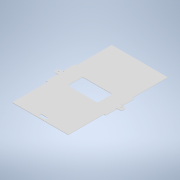
# Autodesk Inventor part: metal_body_forPrint
Saved by Autodesk Inventor 2022 (Build 260153000, 153)
## iProperties
Created: 2024-12-12
Part Number: metal_body_forPrint
Material: Типовые
Document SubType Name: Modeling
Designer: Andrey
Density: 1 g/cm^3
Appearance: По умолчанию
Author: Andrey
Autodesk Inventor part; units mm, degrees
ref_plane "YZ Plane" through (0, 0, 0) normal (1, 0, 0) x (0, 1, 0)
ref_plane "XZ Plane" through (0, 0, 0) normal (0, 1, 0) x (-1, 0, 0)
ref_plane "XY Plane" through (0, 0, 0) normal (0, 0, 1) x (1, 0, 0)
sketch "Эскиз1" plane through (0, 0, 0) normal (0, 1, 0) x (-1, 0, 0)
  line L0 (42.275, -3.8) -> (42.275, -4.36)
  arc A0 (40.675, -5.96) -> (42.275, -4.36) centre (40.675, -4.36) ccw
  line L1 (40.675, -5.96) -> (34.325, -5.96)
  arc A1 (32.725, -4.36) -> (34.325, -5.96) centre (34.325, -4.36) ccw
  line L2 (32.725, -4.36) -> (32.725, -3.8)
  arc A2 (34.325, -2.2) -> (32.725, -3.8) centre (34.325, -3.8) ccw
  line L3 (34.325, -2.2) -> (40.675, -2.2)
  arc A3 (42.275, -3.8) -> (40.675, -2.2) centre (40.675, -3.8) ccw
  arc A4 (55.5, -76.631) -> (57.5, -74.631) centre (55.5, -74.631) ccw
  line L4 (55.5, -76.631) -> (19.5, -76.631)
  arc A5 (17.5, -74.631) -> (19.5, -76.631) centre (19.5, -74.631) ccw
  line L5 (17.5, -74.631) -> (17.5, -58.631)
  arc A6 (19.5, -56.631) -> (17.5, -58.631) centre (19.5, -58.631) ccw
  line L6 (19.5, -56.631) -> (55.5, -56.631)
  arc A7 (57.5, -58.631) -> (55.5, -56.631) centre (55.5, -58.631) ccw
  line L7 (57.5, -58.631) -> (57.5, -74.631)
  line L8 (77.5, -85.631) -> (75, -85.631)
  line L9 (75, -47.631) -> (77.5, -47.631)
  line L10 (75, -47.631) -> (75, 0)
  line L11 (75, 0) -> (0, 0)
  line L12 (0, -47.631) -> (0, 0)
  line L13 (-2.5, -47.631) -> (0, -47.631)
  line L14 (0, -85.631) -> (-2.5, -85.631)
  line L15 (0, -85.631) -> (0, -133.2619)
  line L16 (0, -133.2619) -> (75, -133.2619)
  line L17 (75, -85.631) -> (75, -133.2619)
  line L18 (-0.95, -70.631) -> (-2.5, -70.631)
  line L19 (-2.5, -85.631) -> (-2.5, -70.631)
  line L20 (-2.5, -62.631) -> (-2.5, -47.631)
  line L21 (-2.5, -62.631) -> (-0.95, -62.631)
  line L22 (-0.95, -62.631) -> (-0.95, -63.131)
  line L23 (-4.831, -63.131) -> (-0.95, -63.131)
  line L24 (-4.831, -70.131) -> (-0.95, -70.131)
  line L25 (-0.95, -70.131) -> (-0.95, -70.631)
  arc A8 (-4.831, -63.131) -> (-4.831, -70.131) centre (-4.831, -66.631) ccw
  line L26 (77.5, -70.631) -> (77.5, -85.631)
  line L27 (77.5, -70.631) -> (75.95, -70.631)
  line L28 (75.95, -70.631) -> (75.95, -70.131)
  line L29 (79.831, -70.131) -> (75.95, -70.131)
  arc A9 (79.831, -70.131) -> (79.831, -63.131) centre (79.831, -66.631) ccw
  line L30 (79.831, -63.131) -> (75.95, -63.131)
  line L31 (75.95, -63.131) -> (75.95, -62.631)
  line L32 (75.95, -62.631) -> (77.5, -62.631)
  line L33 (77.5, -47.631) -> (77.5, -62.631)
  arc A10 (55.5, -76.631) -> (57.5, -74.631) centre (55.5, -74.631) ccw
  line L34 (57.5, -74.631) -> (57.5, -58.631)
  arc A11 (57.5, -58.631) -> (55.5, -56.631) centre (55.5, -58.631) ccw
  line L35 (55.5, -56.631) -> (19.5, -56.631)
  arc A12 (19.5, -56.631) -> (17.5, -58.631) centre (19.5, -58.631) ccw
  line L36 (17.5, -58.631) -> (17.5, -74.631)
  arc A13 (17.5, -74.631) -> (19.5, -76.631) centre (19.5, -74.631) ccw
  line L37 (19.5, -76.631) -> (55.5, -76.631)
  circle A14 centre (79.831, -66.631) radius 1
  circle A15 centre (-4.831, -66.631) radius 1
  line L38 (42.275, -4.36) -> (42.275, -3.8)
  arc A16 (42.275, -3.8) -> (40.675, -2.2) centre (40.675, -3.8) ccw
  line L39 (40.675, -2.2) -> (34.325, -2.2)
  arc A17 (34.325, -2.2) -> (32.725, -3.8) centre (34.325, -3.8) ccw
  line L40 (32.725, -3.8) -> (32.725, -4.36)
  arc A18 (32.725, -4.36) -> (34.325, -5.96) centre (34.325, -4.36) ccw
  line L41 (34.325, -5.96) -> (40.675, -5.96)
  arc A19 (40.675, -5.96) -> (42.275, -4.36) centre (40.675, -4.36) ccw
  line L42 (0, 0) -> (0, -47.631)
  line L43 (75, 0) -> (0, 0)
  line L44 (75, -47.631) -> (75, 0)
  line L45 (75, -47.631) -> (77.5, -47.631)
  line L46 (77.5, -62.631) -> (77.5, -47.631)
  line L47 (77.5, -62.631) -> (75.95, -62.631)
  line L48 (75.95, -62.631) -> (75.95, -63.131)
  line L49 (75.95, -63.131) -> (79.831, -63.131)
  arc A20 (79.831, -70.131) -> (79.831, -63.131) centre (79.831, -66.631) ccw
  line L50 (79.831, -70.131) -> (75.95, -70.131)
  line L51 (75.95, -70.131) -> (75.95, -70.631)
  line L52 (75.95, -70.631) -> (77.5, -70.631)
  line L53 (77.5, -85.631) -> (77.5, -70.631)
  line L54 (75, -85.631) -> (77.5, -85.631)
  line L55 (75, -133.2619) -> (75, -85.631)
  line L56 (0, -133.2619) -> (75, -133.2619)
  line L57 (0, -85.631) -> (0, -133.2619)
  line L58 (-2.5, -85.631) -> (0, -85.631)
  line L59 (-2.5, -70.631) -> (-2.5, -85.631)
  line L60 (-2.5, -70.631) -> (-0.95, -70.631)
  line L61 (-0.95, -70.631) -> (-0.95, -70.131)
  line L62 (-4.831, -70.131) -> (-0.95, -70.131)
  arc A21 (-4.831, -63.131) -> (-4.831, -70.131) centre (-4.831, -66.631) ccw
  line L63 (-4.831, -63.131) -> (-0.95, -63.131)
  line L64 (-0.95, -63.131) -> (-0.95, -62.631)
  line L65 (-0.95, -62.631) -> (-2.5, -62.631)
  line L66 (-2.5, -47.631) -> (-2.5, -62.631)
  line L67 (-2.5, -47.631) -> (0, -47.631)
  point P0 (40.675, -5.96)
  point P1 (34.325, -5.96)
  point P2 (34.325, -2.2)
  constraints: 136 end point, 40 point on circle, 22 centre point
extrude "Выдавливание1" add sketch "Эскиз1" along normal blind 0.5
